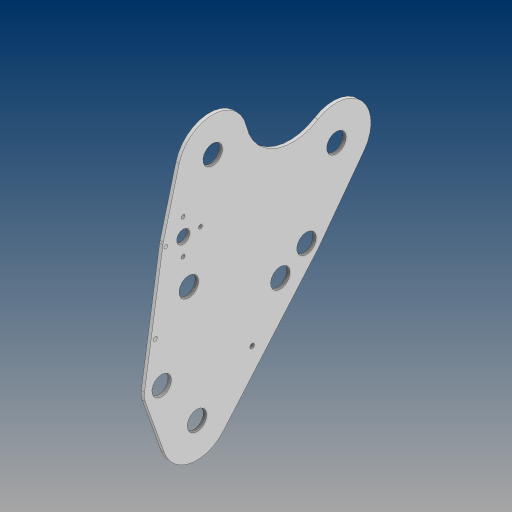
# Autodesk Inventor part: SHOT_1_001_ShooterPlate
Saved by Autodesk Inventor 2024.3 (Build 283343000, 343)
## iProperties
Created: 2024-08-07
Part Number: SHOT_1_001_ShooterPlate
Material: Generic
Document SubType Name: Modeling
Designer: Kenji
Density: 1 g/cm^3
Appearance: Default
Author: Kenji
Autodesk Inventor part; units mm, degrees
ref_plane "YZ Plane" through (0, 0, 0) normal (1, 0, 0) x (0, 1, 0)
ref_plane "XZ Plane" through (0, 0, 0) normal (0, 1, 0) x (-1, 0, 0)
ref_plane "XY Plane" through (0, 0, 0) normal (0, 0, 1) x (1, 0, 0)
sketch "Sketch1" plane through (0, 0, 0) normal (1, 0, 0) x (0, 1, 0)
  line L0 (0, 0) -> (355.6, 0) construction
  line L1 (0, -355.6) -> (0, 0) construction
  line L2 (0, -292.1) -> (279.4, -292.1) construction
  circle A0 centre (377.3626, -124.7533) radius 50.8 construction
  circle A1 centre (301.6507, -306.4608) radius 50.8 construction
  circle A2 centre (339.5066, -215.6071) radius 50.8 construction
  circle A3 centre (301.6507, -306.4608) radius 47.625 construction
  circle A4 centre (377.3626, -124.7533) radius 47.625 construction
  line L3 (377.3626, -124.7533) -> (301.6507, -306.4608) construction
  circle A5 centre (377.3626, -124.7533) radius 14.2875
  circle A6 centre (301.6507, -306.4608) radius 14.2875
  circle A7 centre (226.9166, -89.5837) radius 25.4 construction
  circle A8 centre (170.8921, -224.0415) radius 25.4 construction
  circle A9 centre (170.8921, -224.0415) radius 22.225 construction
  circle A10 centre (226.9166, -89.5837) radius 22.225 construction
  circle A11 centre (226.9166, -89.5837) radius 14.2875
  circle A12 centre (170.8921, -224.0415) radius 14.2875
  line L4 (359.0452, -168.7148) -> (218.3684, -110.0991) construction
  line L5 (319.9681, -262.4993) -> (179.2913, -203.8836) construction
  circle A13 centre (198.8299, -156.9913) radius 50.8 construction
  line L6 (226.9166, -89.5837) -> (170.8921, -224.0415) construction
  circle A14 centre (50.8, -101.6) radius 50.8 construction
  circle A15 centre (193.684, -154.6087) radius 50.8 construction
  line L7 (68.4696, -53.972) -> (211.3536, -106.9807) construction
  line L8 (31.5698, -148.649) -> (176.0144, -202.2367) construction
  circle A16 centre (25.4, -170.0653) radius 25.4 construction
  circle A17 centre (25.4, -170.0653) radius 22.225 construction
  circle A18 centre (25.4, -170.0653) radius 14.2875 construction
  circle A19 centre (121.0331, -49.7674) radius 25.4 construction
  circle A20 centre (121.0331, -49.7674) radius 22.225 construction
  circle A21 centre (121.0331, -49.7674) radius 14.2875
  circle A22 centre (50.8, -101.6) radius 14.2875
  circle A23 centre (41.2055, -25.7462) radius 25.4 construction
  circle A24 centre (41.2055, -25.7462) radius 22.225 construction
  circle A25 centre (41.2055, -25.7462) radius 14.2875 construction
  circle A26 centre (-111.1945, -98.7712) radius 50.8 construction
  circle A27 centre (41.2055, -98.7712) radius 50.8 construction
  line L9 (-111.1945, -47.9712) -> (41.2055, -47.9712) construction
  line L10 (-111.1945, -149.5712) -> (41.2055, -149.5712) construction
  circle A28 centre (294.5226, -81.3968) radius 30 construction
  circle A29 centre (294.5226, -81.3968) radius 25.4 construction
  circle A30 centre (319.9226, -81.3968) radius 2.794
  circle A31 centre (312.4832, -63.4363) radius 2.794
  circle A32 centre (294.5226, -55.9968) radius 2.794
  circle A33 centre (276.5621, -63.4363) radius 2.794
  circle A34 centre (269.1226, -81.3968) radius 2.794
  circle A35 centre (276.5621, -99.3573) radius 2.794
  circle A36 centre (294.5226, -106.7968) radius 2.794
  circle A37 centre (312.4832, -99.3573) radius 2.794
  circle A38 centre (294.5226, -81.3968) radius 9.652
  line L11 (321.1023, -95.308) -> (332.3544, -101.197) construction
  line L12 (264.7402, -85.0034) -> (252.1323, -86.5301) construction
  circle A39 centre (294.5226, -81.3968) radius 9.5504 construction
  circle A40 centre (377.3626, -124.7533) radius 9.5504 construction
  line L13 (381.7912, -116.2917) -> (298.9512, -72.9352) construction
  line L14 (372.934, -133.2148) -> (290.0941, -89.8583) construction
  circle A41 centre (377.3626, -124.7533) radius 14.3256 construction
  circle A42 centre (226.9166, -89.5837) radius 14.3256 construction
  line L15 (223.6556, -103.5332) -> (374.1017, -138.7028) construction
  line L16 (230.1775, -75.6342) -> (380.6236, -110.8038) construction
  circle A43 centre (121.0331, -49.7674) radius 14.3256 construction
  circle A44 centre (226.9166, -89.5837) radius 14.3256 construction
  line L17 (231.9588, -76.1748) -> (126.0753, -36.3585) construction
  line L18 (221.8743, -102.9926) -> (115.9908, -63.1763) construction
  circle A45 centre (170.8921, -224.0415) radius 22.86 construction
  circle A46 centre (195.6336, -262.4886) radius 22.86 construction
  circle A47 centre (195.6336, -262.4886) radius 14.2875
  circle A48 centre (195.6336, -262.4886) radius 9.5504 construction
  line L19 (204.0157, -267.0658) -> (302.9047, -85.974) construction
  line L20 (286.1406, -76.8196) -> (187.2516, -257.9113) construction
  circle A49 centre (104.9224, -182.6351) radius 6.35 construction
  circle A50 centre (104.9224, -182.6351) radius 3.2512
  line L21 (110.3007, -186.0108) -> (149.3787, -210.5385) construction
  arc A51 (388.6007, -174.2946) -> (344.7413, -279.5566) centre (404.0751, -242.5108) ccw
  line L22 (271.3508, -347.2353) -> (181.9987, -280.8371)
  line L23 (390.3161, -75.6326) -> (302.1723, -52.3885)
  line L24 (299.1317, -51.7529) -> (124.9354, -24.669)
  arc A52 (388.6007, -174.2946) -> (390.3161, -75.6326) centre (377.3626, -124.7533) ccw
  arc A53 (271.3508, -347.2353) -> (344.7413, -279.5566) centre (301.6507, -306.4608) ccw
  arc A54 (180.7598, -279.848) -> (181.9987, -280.8371) centre (195.6336, -262.4886) ccw
  arc A55 (302.1723, -52.3885) -> (299.1317, -51.7529) centre (294.5226, -81.3968) ccw
  line L25 (112.55, -25.8259) -> (33.8339, -53.7169)
  line L26 (180.7598, -279.848) -> (17.7471, -140.1765)
  arc A56 (124.9354, -24.669) -> (112.55, -25.8259) centre (121.0331, -49.7674) ccw
  arc A57 (41.9921, -51.5694) -> (17.7471, -140.1765) centre (50.8, -101.6) ccw
  circle A58 centre (184.9724, -40.4298) radius 6.35 construction
  circle A59 centre (184.9724, -40.4298) radius 3.2512
  line L27 (182.7373, -46.3735) -> (179.0171, -56.2667) construction
  point P0 (33.8339, -53.7169)
  dimension "d38" = 50.8
  dimension "d44" = 101.6
  dimension "d82" = 50.8
  dimension "d102" = 12.7
  dimension "d108" = 12.7
  dimension "d13" = 355.6
  dimension "d14" = 355.6
  dimension "d15" = 292.1
  dimension "d29" = 101.6
  dimension "d31" = 3.175
  dimension "d36" = 28.575
  dimension "d39" = 3.175
  dimension "d41" = 28.575
  dimension "d42" = 152.4
  dimension "d43" = 152.4
  dimension "d46" = 279.4
  dimension "d47" = 101.6
  dimension "d48" = 101.6
  dimension "d49" = 152.4
  dimension "d50" = 101.6
  dimension "d51" = 145.6628
  dimension "d59" = 67.38
  dimension "d60" = 28.575
  dimension "d61" = 113.1223
  dimension "d77" = 101.6
  dimension "d78" = 101.6
  dimension "d79" = 152.4
  dimension "d80" = 41.2055
  dimension "d81" = 60
  dimension "d83" = 5.588
  dimension "d86" = 360
  dimension "d88" = 19.304
  dimension "d90" = 12.7
  dimension "d91" = 19.1008
  dimension "d92" = 19.1008
  dimension "d93" = 28.6512
  dimension "d94" = 28.6512
  dimension "d95" = 28.6512
  dimension "d96" = 28.6512
  dimension "d97" = 45.72
  dimension "d99" = 28.575
  dimension "d100" = 19.1008
  dimension "d101" = 206.3329
  dimension "d103" = 6.5024
  dimension "d105" = 46.1377
  dimension "d109" = 6.5024
  dimension "d111" = 56.5611
  constraints: 56 end point, 56 point on circle, 53 centre point, 51 tangent, 23 coincident, 14 equal radius, 9 point on line, 5 concentric, 3 horizontal, 2 horizontal alignment, 2 midpoint, 2 perpendicular, 1 equal length, 1 parallel, 1 vertical alignment, 46 other
  measures "d13" distance of L1.start L0.start
  measures "d14" distance of L0.start L0.end
  measures "d15" distance between parallel lines of L0 L2
  measures "d29" diameter of A1
  measures "d31" radial gap between concentric circles of A1 A3
  measures "d36" diameter of A5
  measures "d41" diameter of A12
  measures "d42" distance of L4.start L4.end
  measures "d43" distance of L5.start L5.end
  measures "d46" distance of L2.start L2.end
  measures "d47" diameter of A14
  measures "d48" diameter of A15
  measures "d49" distance of L7.start L7.end
  measures "d50" distance from line of L0 A14.centre
  measures "d51" distance of L6.start L6.end
  measures "d59" angle of L1 L5
  measures "d60" diameter of A22
  measures "d61" distance of A20.centre point (226.917, -89.584)
  measures "d77" diameter of A26
  measures "d78" diameter of A27
  measures "d79" distance of L10.start L10.end
  measures "d80" distance from line of L1 A23.centre
  measures "d81" diameter of A28
  measures "d83" diameter of A30
  measures "d88" diameter of A38
  measures "d90" distance of L11.start L11.end
  measures "d91" diameter of A39
  measures "d92" diameter of A40
  measures "d93" diameter of A41
  measures "d94" diameter of A42
  measures "d95" diameter of A43
  measures "d96" diameter of A44
  measures "d97" diameter of A45
  measures "d99" diameter of A47
  measures "d100" diameter of A48
  measures "d101" distance of L19.start L19.end
  measures "d103" diameter of A50
  measures "d105" distance of L21.start L21.end
  measures "d109" diameter of A59
  measures "d111" distance of L17.end L27.end
extrude "Extrusion2" add sketch "Sketch1" along normal blind 4.7625 contours A31 | A33 | A35 | A37 | A51 A53 L22 A54 L26 A57 L25 A56 L24 A55 L23 A52
sketch "Sketch2" plane through (4.7625, 0, 0) normal (1, 0, 0) x (0, 0, -1)
  line L0 (25.8259, 112.55) -> (53.7169, 33.8339) projected
  arc A0 (53.7169, 33.8339) -> (140.1765, 17.7471) centre (101.6, 50.8) ccw projected
  line L1 (140.1765, 17.7471) -> (279.848, 180.7598) projected
  arc A1 (279.848, 180.7598) -> (280.8371, 181.9987) centre (262.4886, 195.6336) ccw projected
  line L2 (280.8371, 181.9987) -> (347.2353, 271.3508) projected
  arc A2 (347.2353, 271.3508) -> (279.5566, 344.7413) centre (306.4608, 301.6507) ccw projected
  arc A3 (174.2946, 388.6007) -> (279.5566, 344.7413) centre (242.5108, 404.0751) ccw projected
  arc A4 (174.2946, 388.6007) -> (75.6326, 390.3161) centre (124.7533, 377.3626) ccw projected
  line L3 (75.6326, 390.3161) -> (52.3885, 302.1723) projected
  arc A5 (52.3885, 302.1723) -> (51.7529, 299.1317) centre (81.3968, 294.5226) ccw projected
  line L4 (51.7529, 299.1317) -> (24.669, 124.9354) projected
  arc A6 (24.669, 124.9354) -> (25.8259, 112.55) centre (49.7674, 121.0331) ccw projected
  circle A7 centre (262.4886, 195.6336) radius 14.2875 projected
  circle A8 centre (106.7968, 294.5226) radius 2.794 projected
  circle A9 centre (81.3968, 269.1226) radius 2.794 projected
  circle A10 centre (55.9968, 294.5226) radius 2.794 projected
  circle A11 centre (81.3968, 319.9226) radius 2.794 projected
  circle A12 centre (89.5837, 226.9166) radius 14.2875 projected
  circle A13 centre (40.4298, 184.9724) radius 3.2512 projected
  circle A14 centre (182.6351, 104.9224) radius 3.2512 projected
  circle A15 centre (81.3968, 294.5226) radius 9.652 projected
  circle A16 centre (101.6, 50.8) radius 14.2875 projected
  circle A17 centre (49.7674, 121.0331) radius 14.2875 projected
  circle A18 centre (224.0415, 170.8921) radius 14.2875 projected
  circle A19 centre (306.4608, 301.6507) radius 14.2875 projected
  circle A20 centre (124.7533, 377.3626) radius 14.2875 projected
  point P0 (0, 0)
body "Solid2"
